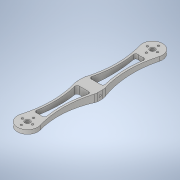
# Autodesk Inventor part: LeverArm
Saved by Autodesk Inventor 2020 (Build 240168000, 168)
## iProperties
Created: 2019-05-25
Part Number: LeverArm
Material: Generic
Document SubType Name: Modeling
Designer: Ryland Lillibridge
Density: 1 g/cm^3
Appearance: Default
Author: Ryland Lillibridge
Autodesk Inventor part; units mm, degrees
ref_plane "YZ Plane" through (0, 0, 0) normal (1, 0, 0) x (0, 1, 0)
sketch "Sketch1" plane through (0, 0, 0) normal (1, 0, 0) x (0, 1, 0)
  circle A0 centre (0, 0) radius 6.35
  line L0 (6.35, 0) -> (6.35, -114.3)
  line L1 (6.35, 0) -> (6.35, 114.3)
  line L2 (6.35, 114.3) -> (0, 114.3)
  arc A1 (-6.3109, 0.7034) -> (0, 114.3) centre (-1025.525, 114.3) ccw
  line L3 (0, 131.3272) -> (0, 114.3) construction
  circle A2 centre (0, 0) radius 1.7145
  line L4 (-6.35, 0) -> (-8.9832, 0)
  line L5 (0, -114.3) -> (6.35, -114.3)
  line L6 (0, -114.3) -> (0, -120.8245) construction
  arc A3 (0, -114.3) -> (-6.3109, -0.7034) centre (-1025.525, -114.3) ccw
  dimension "d0" = 12.7
  dimension "d1" = 114.3
  dimension "d2" = 114.3
  dimension "d3" = 6.35
  dimension "d4" = 3.429
  constraints: 14 end point, 8 point on circle, 5 tangent, 4 centre point, 3 vertical, 2 coincident, 2 horizontal, 1 perpendicular, 1 point on line, 1 symmetric about line
  measures "d0" diameter of A0
  measures "d1" distance of L0.start L0.end
  measures "d2" distance of L0.start L1.end
  measures "d3" distance of L1.end L2.end
  measures "d4" diameter of A2
extrude "Extrusion1" add sketch "Sketch1" along normal blind 31.75
fillet "Fillet1" radius 15.875 4 edges at (31.75, 3.175, 114.3) (0, 3.175, 114.3) (31.75, 3.175, -114.3) (0, 3.175, -114.3)
sketch "Sketch2" plane through (0, 6.35, 98.425) normal (0, 1, 0) x (1, 0, 0)
  arc A0 (0, 0) -> (31.75, 0) centre (15.875, 0) ccw projected
  circle A1 centre (15.875, 0) radius 15.875
  arc A2 (31.75, 196.85) -> (0, 196.85) centre (15.875, 196.85) ccw projected
  circle A3 centre (15.875, 196.85) radius 15.875
  line L0 (15.875, -15.875) -> (15.875, 212.725)
  line L1 (15.875, -15.875) -> (15.875, 98.425)
  line L2 (0, 196.85) -> (0, 99.1284) projected
  line L3 (15.875, 98.425) -> (0, 98.425)
  line L4 (15.875, 98.425) -> (31.75, 98.425)
  line L5 (31.75, 92.075) -> (0, 92.075)
  line L6 (0, 92.075) -> (0, 104.775)
  line L7 (0, 104.775) -> (31.75, 104.775)
  line L8 (31.75, 104.775) -> (31.75, 92.075)
  line L9 (31.75, 92.075) -> (0, 104.775) construction
  line L10 (0, 92.075) -> (31.75, 104.775) construction
  arc A4 (0.6373, 4.453) -> (0, 92.075) centre (-145.6441, 47.2023) ccw
  arc A5 (31.75, 92.075) -> (31.1127, 4.453) centre (177.3941, 47.2023) ccw
  line L11 (0, 196.85) -> (0, 0) projected
  line L12 (0, 0) -> (0, 92.075)
  line L13 (31.75, 97.7216) -> (31.75, 0) projected
  line L14 (31.75, 0) -> (31.75, 92.075)
  dimension "d8" = 114.3
  dimension "d9" = 31.75
  dimension "d10" = 12.7
  dimension "d11" = 152.4
  dimension "d12" = 152.4
  constraints: 24 end point, 12 point on circle, 4 centre point, 3 midpoint, 2 coincident, 2 parallel, 2 tangent, 1 horizontal, 1 perpendicular
  measures "d8" distance of L0.start L1.end
  measures "d9" distance of L6.end L7.end
  measures "d10" distance of L5.end L6.end
  measures "d11" radius of A4
  measures "d12" radius of A5
extrude "Extrusion2" cut sketch "Sketch2" against normal blind 20.6375 contours L11 A4 A1 | A1 A5 L13
sketch "Sketch3" plane through (15.875, 6.35, -98.425) normal (0, 1, 0) x (1, 0, 0)
  line L0 (-15.875, 130.175) -> (15.875, 130.175)
  line L1 (15.875, 130.175) -> (15.875, -98.425)
  line L2 (15.875, -98.425) -> (-15.875, -98.425)
  line L3 (-15.875, -98.425) -> (-15.875, 130.175)
  arc A0 (15.875, 0) -> (-15.875, 0) centre (0, 0) ccw projected
  line L4 (-15.875, 130.175) -> (15.875, -98.425) construction
  line L5 (15.875, 130.175) -> (-15.875, -98.425) construction
  point P0 (-15.875, -98.425)
  point P1 (-15.875, -99.1284)
  point P2 (15.875, -99.1284)
  point P3 (0, 15.875)
  dimension "d15" = 31.75
  dimension "d16" = 228.6
  constraints: 12 end point, 2 midpoint, 2 parallel, 1 horizontal, 1 perpendicular, 1 point on circle
  measures "d15" distance of L1.end L2.end
  measures "d16" distance of L0.end L1.end
extrude "Extrusion3" cut sketch "Sketch3" against normal blind 25.4 contours A0 L1 L2 L3
sketch "Sketch4" plane through (15.875, 6.35, 98.425) normal (0, 1, 0) x (1, 0, 0)
  arc A0 (15.2377, 4.453) -> (-15.2377, 4.453) centre (0, 0) ccw construction
  arc A1 (15.875, 92.075) -> (15.2377, 4.453) centre (161.5191, 47.2023) ccw construction
  arc A2 (-15.2377, 4.453) -> (-15.875, 92.075) centre (-161.5191, 47.2023) ccw construction
  line L0 (-12.5559, 92.075) -> (-15.875, 92.075) construction
  arc A3 (8.9391, 16.8224) -> (-8.9391, 16.8224) centre (0, 0) ccw
  arc A4 (11.6362, 88.9) -> (8.9391, 16.8224) centre (161.5191, 47.2023) ccw
  arc A5 (-8.9391, 16.8224) -> (-11.6362, 88.9) centre (-161.5191, 47.2023) ccw
  line L1 (0, 92.075) -> (0, 88.9) construction
  line L2 (0, 88.9) -> (-11.6362, 88.9)
  line L3 (-11.6362, 88.9) -> (11.6362, 88.9)
  line L4 (11.6362, 88.9) -> (-11.6362, 88.9)
  point P0 (-15.875, 98.425)
  dimension "d19" = 15.875
  dimension "d20" = 152.4
  dimension "d21" = 152.4
  dimension "d22" = 31.75
  dimension "d23" = 38.1
  dimension "d24" = 311.15
  dimension "d25" = 311.15
  dimension "d26" = 3.175
  constraints: 11 point on circle, 10 end point, 4 centre point, 3 coincident, 3 horizontal, 1 vertical
  measures "d19" radius of A0
  measures "d20" radius of A1
  measures "d21" radius of A2
  measures "d22" distance of A1.start L0.end
  measures "d23" diameter of A3
  measures "d24" diameter of A4
  measures "d25" diameter of A5
  measures "d26" distance of L1.start L1.end
extrude "Extrusion4" cut sketch "Sketch4" against normal blind 25.4
fillet "Fillet2" radius 15.875 2 edges at (31.75, 0.3263, 6.35) (0, 0.3263, 6.35)
mirror "Mirror1" about plane through (31.75, 6.35, 0) normal (0, 0, -1)
sketch "Sketch5" plane through (15.875, 6.35, 98.425) normal (0, 1, 0) x (1, 0, 0)
  circle A0 centre (0, 0) radius 15.875 construction
  arc A1 (15.2377, 192.397) -> (-15.2377, 192.397) centre (0, 196.85) ccw projected
  circle A2 centre (0, 196.85) radius 15.875 construction
  circle A3 centre (0, 0) radius 9.5 construction
  circle A4 centre (0, 0) radius 8 construction
  circle A5 centre (0, 196.85) radius 9.5 construction
  circle A6 centre (0, 196.85) radius 8 construction
  circle A7 centre (0, 187.35) radius 1.5875
  circle A8 centre (0, 206.35) radius 1.5875
  circle A9 centre (-8, 196.85) radius 1.5875
  circle A10 centre (8, 196.85) radius 1.5875
  circle A11 centre (0, 9.5) radius 1.5875
  circle A12 centre (0, -9.5) radius 1.5875
  circle A13 centre (-8, 0) radius 1.5875
  circle A14 centre (8, 0) radius 1.5875
  circle A15 centre (0, 0) radius 3.175
  circle A16 centre (0, 196.85) radius 3.175
  point P0 (-15.875, 98.425)
  dimension "d30" = 19
  dimension "d31" = 16
  dimension "d32" = 19
  dimension "d33" = 16
  dimension "d34" = 3.175
  dimension "d35" = 3.175
  dimension "d36" = 3.175
  dimension "d37" = 3.175
  dimension "d38" = 3.175
  dimension "d39" = 3.175
  dimension "d40" = 3.175
  dimension "d41" = 3.175
  dimension "d42" = 6.35
  dimension "d43" = 6.35
  constraints: 16 centre point, 8 point on circle, 7 coincident
  measures "d30" diameter of A3
  measures "d31" diameter of A4
  measures "d32" diameter of A5
  measures "d33" diameter of A6
  measures "d34" diameter of A7
  measures "d35" diameter of A8
  measures "d36" diameter of A9
  measures "d37" diameter of A10
  measures "d38" diameter of A11
  measures "d39" diameter of A12
  measures "d40" diameter of A13
  measures "d41" diameter of A14
  measures "d42" diameter of A15
  measures "d43" diameter of A16
extrude "Extrusion5" cut sketch "Sketch5" against normal blind 25.4
ref_plane "Work Plane1" through (15.875, 1.35, 98.425) normal (0, 1, 0) x (1, 0, 0)
sketch "Sketch8" plane through (15.875, 1.35, 98.425) normal (0, 1, 0) x (1, 0, 0)
  circle A0 centre (8, 196.85) radius 1.5875 projected
  circle A1 centre (8, 196.85) radius 3
  circle A2 centre (0, 206.35) radius 1.5875 projected
  circle A3 centre (0, 206.35) radius 3
  circle A4 centre (-8, 196.85) radius 1.5875 projected
  circle A5 centre (-8, 196.85) radius 3
  circle A6 centre (0, 187.35) radius 1.5875 projected
  circle A7 centre (0, 187.35) radius 3
  circle A8 centre (0, 9.5) radius 1.5875 projected
  circle A9 centre (0, 9.5) radius 3
  circle A10 centre (8, 0) radius 1.5875 projected
  circle A11 centre (8, 0) radius 3
  circle A12 centre (-8, 0) radius 1.5875 projected
  circle A13 centre (-8, 0) radius 3
  circle A14 centre (0, -9.5) radius 1.5875 projected
  circle A15 centre (0, -9.5) radius 3
  point P0 (-15.875, 98.425)
  dimension "d47" = 6
  dimension "d48" = 6
  dimension "d49" = 6
  dimension "d50" = 6
  dimension "d51" = 6
  dimension "d52" = 6
  dimension "d53" = 6
  dimension "d54" = 6
  constraints: 8 centre point, 8 coincident
  measures "d47" diameter of A1
  measures "d48" diameter of A3
  measures "d49" diameter of A5
  measures "d50" diameter of A7
  measures "d51" diameter of A9
  measures "d52" diameter of A11
  measures "d53" diameter of A13
  measures "d54" diameter of A15
extrude "Extrusion6" cut sketch "Sketch8" against normal blind 25.4 contours A0 | A1 | A2 | A3 | A4 | A5 | A6 | A7 | A8 | A9 | A11 | A12 | A13 | A14 | A15
fillet "Fillet3" radius 1 8 edges at (21.0034, -0.1367, 97.5568) (13.0035, -0.0256, 107.0564) (5.0034, -0.1367, 97.5568) (13.0031, -0.3358, 88.0578) (12.8751, -0.3146, -88.9) (21.0033, -0.1098, -99.2929) (13.0035, -0.0148, -108.7935) (4.8751, -0.1233, -98.3999)
fillet "Fillet4" radius 1 2 edges at (12.7, 6.35, -98.425) (12.7, 6.35, 98.425)
fillet "Fillet5" radius 3.175 8 edges at (24.8141, 2.9143, 81.6026) (6.9359, 2.9143, 81.6026) (27.5112, 0.4918, 9.525) (4.2388, 0.4918, 9.525) (27.5112, 0.4918, -9.525) (4.2388, 0.4918, -9.525) (6.9359, 2.9143, -81.6026) (24.8141, 2.9143, -81.6026)
ref_plane "Work Plane2" through (15.875, 0, 98.425) normal (0, 1, 0) x (1, 0, 0)
sketch "Sketch9" plane through (15.875, 0, 98.425) normal (0, 1, 0) x (1, 0, 0)
  line L0 (18.7215, 180.9942) -> (-17.0964, 180.9942)
  line L1 (-17.0964, 180.9942) -> (-17.0964, 213.6283)
  line L2 (-17.0964, 213.6283) -> (18.7215, 213.6283)
  line L3 (18.7215, 213.6283) -> (18.7215, 180.9942)
  line L4 (-15.875, 99.1284) -> (15.875, 99.1284) projected
  line L5 (13.6091, 97.7216) -> (13.6091, 99.1284)
  line L6 (13.6091, 98.425) -> (20.0135, 98.425)
  line L7 (18.7215, 15.8558) -> (-17.0964, 15.8558)
  line L8 (-17.0964, 15.8558) -> (-17.0964, -16.7783)
  line L9 (-17.0964, -16.7783) -> (18.7215, -16.7783)
  line L10 (18.7215, -16.7783) -> (18.7215, 15.8558)
  point P0 (-15.875, 98.425)
  dimension "d63" = 32.6341
  constraints: 20 end point, 4 symmetric about line, 2 horizontal, 2 parallel, 1 midpoint, 1 perpendicular, 1 point on line, 1 vertical
  measures "d63" distance between parallel lines of L0 L2
extrude "Extrusion7" [suppressed]
body "Solid1"
